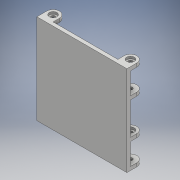
# Autodesk Inventor part: MecanumPlate_FEA
Saved by Autodesk Inventor 2018 (Build 220112000, 112)
## iProperties
Created: 2017-09-19
Part Number: MecanumPlate_FEA
Material: Generic
Document SubType Name: Modeling
Designer: P136265
Density: 1 g/cm^3
Appearance: Default
Author: P136265
Autodesk Inventor part; units mm, degrees
ref_plane "YZ Plane" through (0, 0, 0) normal (1, 0, 0) x (0, 1, 0)
ref_plane "XZ Plane" through (0, 0, 0) normal (0, 1, 0) x (-1, 0, 0)
sketch "Sketch1" plane through (0, 0, 0) normal (0, 0, 1) x (1, 0, 0)
  line L0 (-250, -10) -> (250, -10)
  line L1 (250, -10) -> (250, 10)
  line L2 (250, 10) -> (-250, 10)
  line L3 (-250, 10) -> (-250, -10)
  line L4 (-250, -10) -> (250, 10) construction
  line L5 (250, -10) -> (-250, 10) construction
  point P0 (0, 0)
  dimension "d0" = 500
  dimension "d1" = 20
  constraints: 12 end point, 2 midpoint, 2 parallel, 1 horizontal, 1 perpendicular
  measures "d0" distance of L2.end L1.end
  measures "d1" distance of L1.end L0.end
extrude "Extrusion1" add sketch "Sketch1" along normal mid plane 500
sketch "Sketch2" plane through (0, 0, 250) normal (0, 0, 1) x (1, 0, 0)
  arc A0 (-180, 45) -> (-250, 45) centre (-215, 45) ccw
  line L0 (250, 10) -> (-250, 10) construction
  circle A1 centre (-215, 45) radius 11
  line L1 (-250, 45) -> (-250, 0)
  line L2 (-180, 45) -> (-180, 0)
  line L3 (-180, 0) -> (-250, 0)
  point P0 (0, 0)
  dimension "d4" = 70
  dimension "d5" = 215
  dimension "d6" = 45
  dimension "d7" = 22
  dimension "d9" = 10
  constraints: 6 end point, 2 centre point, 2 point on circle, 2 tangent, 2 vertical, 1 coincident, 1 perpendicular
  measures "d4" diameter of A0
  measures "d5" horizontal distance of point (0, 0) A0.centre
  measures "d6" vertical distance of point (0, 0) A0.centre
  measures "d7" diameter of A1
  measures "d9" distance between parallel lines of L3 L0
extrude "Extrusion2" add sketch "Sketch2" against normal blind 20
ref_plane "Work Plane1" through (0, 0, 90) normal (0, 0, 1) x (1, 0, 0)
sketch "Sketch3" plane through (0, 0, 90) normal (0, 0, 1) x (1, 0, 0)
  arc A0 (-180, 45) -> (-250, 45) centre (-215, 45) ccw construction
  circle A1 centre (-215, 45) radius 11 construction
  line L0 (-180, 45) -> (-180, 10) construction
  line L1 (-250, 45) -> (-250, -10) construction
  circle A2 centre (-215, 45) radius 11
  arc A3 (-180, 45) -> (-250, 45) centre (-215, 45) ccw
  line L2 (-250, 45) -> (-250, 0)
  line L3 (-180, 45) -> (-180, 0)
  line L4 (-180, 0) -> (-250, 0)
  point P0 (0, 0)
  constraints: 6 end point, 4 tangent, 3 point on line, 2 centre point, 2 coincident, 2 concentric, 2 point on circle, 1 perpendicular
extrude "Extrusion3" add sketch "Sketch3" along normal blind 20
sketch "Sketch4" plane through (0, 0, 250) normal (0, 0, 1) x (1, 0, 0)
  circle A0 centre (-215, 45) radius 11 construction
  circle A1 centre (-215, 45) radius 21
  point P0 (0, 0)
  dimension "d15" = 42
  constraints: 1 centre point, 1 coincident
  measures "d15" diameter of A1
extrude "Extrusion4" cut sketch "Sketch4" against normal blind 12
sketch "Sketch5" plane through (0, 0, 90) normal (0, 0, -1) x (-1, 0, 0)
  circle A0 centre (215, 45) radius 11 construction
  circle A1 centre (215, 45) radius 21
  point P0 (0, 0)
  dimension "d18" = 42
  constraints: 1 centre point, 1 coincident
  measures "d18" diameter of A1
extrude "Extrusion5" cut sketch "Sketch5" against normal blind 12
sketch "Sketch6" plane through (0, 0, 250) normal (0, 0, 1) x (1, 0, 0)
  arc A0 (250, 45) -> (180, 45) centre (215, 45) ccw
  circle A1 centre (215, 45) radius 11
  line L0 (180, 45) -> (180, 0)
  line L1 (180, 0) -> (250, 0)
  line L2 (250, 0) -> (250, 45)
  point P0 (0, 0)
  dimension "d21" = 70
  dimension "d22" = 215
  dimension "d23" = 45
  dimension "d24" = 22
  dimension "d25" = 0
  constraints: 6 end point, 2 centre point, 2 perpendicular, 2 point on circle, 2 tangent, 1 coincident, 1 vertical
  measures "d21" diameter of A0
  measures "d22" horizontal distance of point (0, 0) A0.centre
  measures "d23" vertical distance of point (0, 0) A0.centre
  measures "d24" diameter of A1
  measures "d25" distance from line of point (0, 0) L1
extrude "Extrusion6" add sketch "Sketch6" against normal blind 20
sketch "Sketch7" plane through (0, 0, 90) normal (0, 0, 1) x (1, 0, 0)
  arc A0 (250, 45) -> (180, 45) centre (215, 45) ccw construction
  circle A1 centre (215, 45) radius 11 construction
  arc A2 (250, 45) -> (180, 45) centre (215, 45) ccw
  circle A3 centre (215, 45) radius 11 projected
  circle A4 centre (215, 45) radius 11
  line L0 (250, 45) -> (250, 10) projected
  line L1 (250, 45) -> (250, 0)
  line L2 (250, 0) -> (250, 0)
  arc A5 (250, 45) -> (180, 45) centre (215, 45) ccw projected
  line L3 (250, 0) -> (250, 45)
  line L4 (180, 45) -> (180, 0)
  line L5 (180, 0) -> (250, 0)
  point P0 (0, 0)
  dimension "d28" = 22
  dimension "d29" = 45
  constraints: 10 end point, 3 perpendicular, 2 centre point, 2 coincident, 2 point on circle, 2 tangent, 1 collinear, 1 vertical
  measures "d28" diameter of A4
  measures "d29" distance from line of L0.start L2
extrude "Extrusion7" add sketch "Sketch7" along normal blind 20
sketch "Sketch8" plane through (0, 0, 250) normal (0, 0, 1) x (1, 0, 0)
  circle A0 centre (215, 45) radius 11 construction
  circle A1 centre (215, 45) radius 21
  point P0 (0, 0)
  dimension "d32" = 42
  constraints: 1 centre point, 1 coincident
  measures "d32" diameter of A1
extrude "Extrusion8" cut sketch "Sketch8" against normal blind 12
sketch "Sketch9" plane through (0, 0, 90) normal (0, 0, -1) x (-1, 0, 0)
  circle A0 centre (-215, 45) radius 11 construction
  circle A1 centre (-215, 45) radius 21
  point P0 (0, 0)
  dimension "d35" = 42
  constraints: 1 centre point, 1 coincident
  measures "d35" diameter of A1
extrude "Extrusion9" cut sketch "Sketch9" against normal blind 12
sketch "Sketch10" plane through (0, 0, -250) normal (0, 0, -1) x (-1, 0, 0)
  arc A0 (-180, 45) -> (-250, 45) centre (-215, 45) ccw construction
  line L0 (-180, 45) -> (-180, 10) construction
  line L1 (-250, 10) -> (-250, 45) construction
  line L2 (250, 10) -> (-250, 10) construction
  circle A1 centre (-215, 45) radius 11 construction
  arc A2 (-180, 45) -> (-250, 45) centre (-215, 45) ccw
  arc A3 (-180, 45) -> (-250, 45) centre (-215, 45) ccw projected
  circle A4 centre (-215, 45) radius 11
  line L3 (-250, 45) -> (-250, 10)
  line L4 (-250, -10) -> (-250, 45) construction
  line L5 (-180, 10) -> (-180, 45)
  line L6 (-250, 10) -> (-180, 10)
  point P0 (0, 0)
  dimension "d38" = 22
  constraints: 6 end point, 2 centre point, 2 coincident, 2 point on circle, 1 collinear, 1 parallel, 1 perpendicular, 1 point on line
  measures "d38" diameter of A4
extrude "Extrusion10" add sketch "Sketch10" against normal blind 20
sketch "Sketch11" plane through (0, 0, -250) normal (0, 0, -1) x (-1, 0, 0)
  arc A0 (250, 45) -> (180, 45) centre (215, 45) ccw construction
  circle A1 centre (215, 45) radius 11 construction
  arc A2 (250, 45) -> (180, 45) centre (215, 45) ccw
  arc A3 (250, 45) -> (180, 45) centre (215, 45) ccw projected
  circle A4 centre (215, 45) radius 11
  line L0 (180, 45) -> (180, 10) projected
  line L1 (180, 10) -> (250, 10) projected
  line L2 (180, 45) -> (180, 10)
  line L3 (180, 10) -> (250, 10)
  line L4 (250, 10) -> (250, 45)
  point P0 (0, 0)
  dimension "d41" = 22
  constraints: 6 end point, 2 centre point, 2 coincident, 2 perpendicular, 2 point on circle, 1 collinear, 1 concentric, 1 point on line
  measures "d41" diameter of A4
extrude "Extrusion11" add sketch "Sketch11" against normal blind 20
ref_plane "Work Plane2" through (0, 0, -90) normal (0, 0, 1) x (1, 0, 0)
sketch "Sketch12" plane through (0, 0, -90) normal (0, 0, 1) x (1, 0, 0)
  arc A0 (250, 45) -> (180, 45) centre (215, 45) ccw construction
  circle A1 centre (215, 45) radius 11 construction
  arc A2 (250, 45) -> (180, 45) centre (215, 45) ccw
  arc A3 (250, 45) -> (180, 45) centre (215, 45) ccw projected
  circle A4 centre (215, 45) radius 11
  line L0 (250, 10) -> (180, 10) projected
  line L1 (250, 45) -> (250, 10)
  line L2 (250, 10) -> (180, 10)
  line L3 (180, 10) -> (180, 45)
  point P0 (0, 0)
  constraints: 6 end point, 3 point on circle, 2 centre point, 2 coincident, 1 collinear, 1 concentric, 1 perpendicular, 1 vertical
extrude "Extrusion12" add sketch "Sketch12" against normal blind 20
sketch "Sketch13" plane through (0, 0, -250) normal (0, 0, -1) x (-1, 0, 0)
  circle A0 centre (-215, 45) radius 11 construction
  circle A1 centre (-215, 45) radius 21
  point P0 (0, 0)
  dimension "d47" = 42
  constraints: 1 centre point, 1 coincident
  measures "d47" diameter of A1
extrude "Extrusion13" cut sketch "Sketch13" against normal blind 12
sketch "Sketch14" plane through (0, 0, -90) normal (0, 0, 1) x (1, 0, 0)
  circle A0 centre (215, 45) radius 11 construction
  circle A1 centre (215, 45) radius 21
  point P0 (0, 0)
  dimension "d50" = 42
  constraints: 1 centre point, 1 coincident
  measures "d50" diameter of A1
extrude "Extrusion14" cut sketch "Sketch14" against normal blind 12
sketch "Sketch15" plane through (0, 0, -90) normal (0, 0, 1) x (1, 0, 0)
  arc A0 (-180, 45) -> (-250, 45) centre (-215, 45) ccw projected
  arc A1 (-180, 45) -> (-250, 45) centre (-215, 45) ccw
  arc A2 (-180, 45) -> (-250, 45) centre (-215, 45) ccw construction
  circle A3 centre (-215, 45) radius 11 construction
  circle A4 centre (-215, 45) radius 11
  line L0 (-180, 45) -> (-180, 10) projected
  line L1 (-180, 45) -> (-180, 10)
  line L2 (-250, 10) -> (-180, 10) projected
  line L3 (-180, 10) -> (-250, 10)
  line L4 (-250, 10) -> (-250, 45)
  point P0 (0, 0)
  dimension "d53" = 22
  constraints: 6 end point, 3 centre point, 3 coincident, 2 collinear, 2 concentric, 2 point on circle, 1 perpendicular, 1 point on line
  measures "d53" diameter of A3
extrude "Extrusion15" add sketch "Sketch15" against normal blind 20
sketch "Sketch16" plane through (0, 0, -250) normal (0, 0, -1) x (-1, 0, 0)
  circle A0 centre (215, 45) radius 11 construction
  circle A1 centre (215, 45) radius 21
  point P0 (0, 0)
  dimension "d56" = 42
  constraints: 1 centre point, 1 coincident
  measures "d56" diameter of A1
extrude "Extrusion16" cut sketch "Sketch16" against normal blind 12
sketch "Sketch17" plane through (0, 0, -90) normal (0, 0, 1) x (1, 0, 0)
  circle A0 centre (-215, 45) radius 11 construction
  circle A1 centre (-215, 45) radius 21
  point P0 (0, 0)
  dimension "d59" = 42
  constraints: 1 centre point, 1 coincident
  measures "d59" diameter of A1
extrude "Extrusion17" cut sketch "Sketch17" against normal blind 12
body "Solid1"
